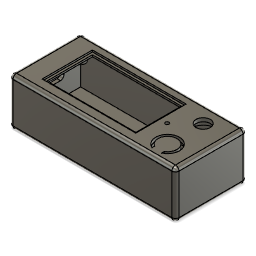
Case (Autodesk Fusion 360 design; units mm, degrees)
Autodesk Fusion 360 part; units mm, degrees
sketch "Sketch1" plane through (0, 0, 0) normal (0, 1, 0) x (1, 0, 0) in component "Toppen"
  line L0 (33.5, -15) -> (-33.5, -15)
  line L1 (-35, -13.5) -> (-35, 13.5)
  line L2 (-33.5, 15) -> (33.5, 15)
  line L3 (35, 13.5) -> (35, -13.5)
  line L4 (35, -15) -> (-35, 15) construction
  line L5 (-35, -15) -> (35, 15) construction
  arc A0 (35, 13.5) -> (33.5, 15) centre (33.5, 13.5) ccw
  arc A1 (-33.5, 15) -> (-35, 13.5) centre (-33.5, 13.5) ccw
  arc A2 (-35, -13.5) -> (-33.5, -15) centre (-33.5, -13.5) ccw
  arc A3 (33.5, -15) -> (35, -13.5) centre (33.5, -13.5) ccw
  dimension "d1" = 70
  dimension "d2" = 30
  dimension "d3" = 1.5
  constraint horizontal L0
  constraint perpendicular L0 L1
  constraint parallel L0 L2
  constraint parallel L1 L3
  constraint coincident L4 origin
  constraint coincident L5 origin
  constraint coincident L5.end L3
  constraint coincident L5.end L2
  constraint tangent L3 A0
  constraint tangent L2 A0
  constraint coincident L4.end L2
  constraint coincident L4.end L1
  constraint tangent L2 A1
  constraint tangent L1 A1
  constraint equal A0 A1
  constraint coincident L5.start L1
  constraint coincident L5.start L0
  constraint tangent L1 A2
  constraint tangent L0 A2
  constraint equal A0 A2
  constraint coincident L4.start L3
  constraint coincident L4.start L0
  constraint tangent L3 A3
  constraint tangent L0 A3
  constraint equal A0 A3
  measures "d1" distance of L4.end L5.end
  measures "d2" distance of L4.start L5.end
  measures "d3" radius of A0
extrude "Extrude1" add sketch "Sketch1" against normal blind 18.5 makes body 1 in component "Toppen"
move_body "Move1" bodies 1 to x (1, 0, 0) y (0, 1, 0) z (0, 0, 1) at (0, 15, 0) in component "Toppen"
shell "Shell1" thickness 1.5 removed faces 1 at (11.1667, -3.5, 5) on bodies 1 in component "Toppen"
extrude "Extrude1'" add sketch "Sketch1" along normal blind 1.5 separate body makes body 2 in component "Botten"
sketch "Sketch1 (2)" plane through (0, 20, 0) normal (0, 1, 0) x (-1, 0, 0) in component "Botten"
  arc A0 (35, 13.5) -> (33.5, 15) centre (33.5, 13.5) ccw
  line L0 (33.5, 15) -> (-33.5, 15)
  arc A1 (-33.5, 15) -> (-35, 13.5) centre (-33.5, 13.5) ccw
  line L1 (-35, 13.5) -> (-35, -13.5)
  arc A2 (-35, -13.5) -> (-33.5, -15) centre (-33.5, -13.5) ccw
  line L2 (-33.5, -15) -> (33.5, -15)
  arc A3 (33.5, -15) -> (35, -13.5) centre (33.5, -13.5) ccw
  line L3 (35, -13.5) -> (35, 13.5)
  line L4 (35, 0) -> (29, 0) construction
  line L5 (29, 0) -> (29, 8.75) construction
  line L6 (29, 8.75) -> (-16.7, 8.75) construction
  line L7 (-16.7, 8.75) -> (-16.7, -9.05) construction
  line L8 (-16.7, -9.05) -> (29, -9.05) construction
  line L9 (29, -9.05) -> (29, 8.75) construction
  circle A4 centre (29, -9.05) radius 2
  circle A5 centre (29, 8.75) radius 2
  circle A6 centre (-16.7, -9.05) radius 2
  circle A7 centre (-16.7, 8.75) radius 2
  line L10 (35, 0) -> (31.5, 0) construction
  line L11 (31.5, 0) -> (31.5, 11.5) construction
  line L12 (31.5, 11.5) -> (-19.5, 11.5) construction
  line L13 (-19.5, 11.5) -> (-19.5, -11.5) construction
  line L14 (-19.5, -11.5) -> (31.5, -11.5) construction
  line L15 (31.5, -11.5) -> (31.5, 11.5) construction
  line L16 (31.5, -11.5) -> (24, -11.5) construction
  line L17 (24, -11.5) -> (24, -9) construction
  line L18 (24, -9) -> (31.5, -9) construction
  line L19 (31.5, -9) -> (31.5, -11.5) construction
  line L20 (24, -9) -> (-11.5, -9) construction
  line L21 (-11.5, -9) -> (-11.5, 8.2) construction
  line L22 (-11.5, 8.2) -> (24, 8.2) construction
  line L23 (24, 8.2) -> (24, -9) construction
  line L24 (-11.5, 8.2) -> (24, -9) construction
  line L25 (-11.5, -9) -> (24, 8.2) construction
  line L26 (25, 9.2) -> (-12.5, 9.2)
  line L27 (-12.5, 9.2) -> (-12.5, -10)
  line L28 (-12.5, -10) -> (25, -10)
  line L29 (25, -10) -> (25, 9.2)
  line L30 (25, 9.2) -> (-12.5, -10) construction
  line L31 (-12.5, 9.2) -> (25, -10) construction
  line L32 (26, 10.2) -> (-13.5, 10.2)
  line L33 (-13.5, 10.2) -> (-13.5, -11)
  line L34 (-13.5, -11) -> (26, -11)
  line L35 (26, -11) -> (26, 10.2)
  line L36 (26, 10.2) -> (-13.5, -11) construction
  line L37 (-13.5, 10.2) -> (26, -11) construction
  line L38 (-16.7, -9.05) -> (-16.7, -0.05) construction
  line L39 (-16.7, -0.05) -> (-16.5, -0.05) construction
  circle A8 centre (-16.5, -0.05) radius 0.75
  point P0 (6.25, -0.4)
  point P1 (6.25, -0.4)
  dimension "d11" = 6
  dimension "d12" = 8.75
  dimension "d13" = 45.7
  dimension "d14" = 17.8
  dimension "d15" = 4
  dimension "d16" = 4
  dimension "d17" = 4
  dimension "d18" = 4
  dimension "d19" = 3.5
  dimension "d20" = 11.5
  dimension "d21" = 51
  dimension "d22" = 23
  dimension "d23" = 7.5
  dimension "d24" = 2.5
  dimension "d25" = 35.5
  dimension "d26" = 17.2
  dimension "d27" = 37.5
  dimension "d28" = 19.2
  dimension "d29" = 39.5
  dimension "d30" = 21.2
  dimension "d43" = 9
  dimension "d44" = 0.2
  dimension "d45" = 1.5
  constraint midpoint L3 L4.start
  constraint perpendicular L3 L4
  constraint perpendicular L4 L5
  constraint horizontal L6
  constraint vertical L7
  constraint horizontal L8
  constraint vertical L9
  constraint coincident L8.end L9.start
  constraint coincident L5.end L6.start
  constraint coincident L7.end L8.start
  constraint coincident L6.end L7.start
  constraint perpendicular L3 L10
  constraint perpendicular L10 L11
  constraint horizontal L12
  constraint vertical L13
  constraint horizontal L14
  constraint vertical L15
  constraint vertical L17
  constraint perpendicular L16 L17
  constraint horizontal L18
  constraint parallel L17 L19
  constraint horizontal L20
  constraint vertical L21
  constraint horizontal L22
  constraint vertical L23
  constraint horizontal L26
  constraint perpendicular L26 L27
  constraint parallel L26 L28
  constraint parallel L27 L29
  constraint coincident L30 P1
  constraint coincident L31 P1
  constraint midpoint L25 P1
  constraint horizontal L32
  constraint perpendicular L32 L33
  constraint parallel L32 L34
  constraint parallel L33 L35
  constraint coincident L36 P1
  constraint coincident L37 P1
  constraint coincident P1 P0
  constraint perpendicular L8 L38
  constraint perpendicular L38 L39
  constraint coincident L39.end A8.centre
  measures "d11" distance of L4.start L4.end
  measures "d12" distance of L4.end L5.end
  measures "d13" distance of L5.end L6.end
  measures "d14" distance of L5.end L8.end
  measures "d15" diameter of A4
  measures "d16" diameter of A5
  measures "d17" diameter of A6
  measures "d18" diameter of A7
  measures "d19" distance of L4.start L10.end
  measures "d20" distance of L10.end L11.end
  measures "d21" distance of L11.end L12.end
  measures "d22" distance of L11.end L14.end
  measures "d23" distance of L14.end L16.end
  measures "d24" distance of L14.end L18.end
  measures "d25" distance of L17.end L20.end
  measures "d26" distance of L17.end L22.end
  measures "d27" distance of L27.end L28.end
  measures "d28" distance of L26.end L27.end
  measures "d29" distance of L33.end L34.end
  measures "d30" distance of L32.end L33.end
  measures "d43" distance of L7.end L38.end
  measures "d44" distance of L38.end L39.end
  measures "d45" diameter of A8
extrude "Extrude3" cut sketch "Sketch1 (2)" against normal blind 1.5 contours L26 L27 L28 L29 sketch seen with x (1, 0, 0) y (0, 1, 0) z (0, 0, 1) at (0, -5, 0) bodies 1 in component "Toppen"
extrude "Extrude4" cut sketch "Sketch1 (2)" against normal blind 0.75 contours L32 L33 L34 L35 sketch seen with x (1, 0, 0) y (0, 1, 0) z (0, 0, 1) at (0, -5, 0) bodies 1 in component "Toppen"
extrude "Extrude5" add sketch "Sketch1 (2)" against normal blind 4.5 contours A4 | A5 | A6 | A7 sketch seen with x (1, 0, 0) y (0, 1, 0) z (0, 0, 1) at (0, -5, 0) bodies 1 in component "Toppen"
sketch "Sketch2" plane through (0, 10.5, 0) normal (0, -1, 0) x (1, 0, 0) in component "Toppen"
  circle A0 centre (-29, 8.75) radius 2
  circle A1 centre (-29, 8.75) radius 0.75
  dimension "d37" = 1.5
  constraint concentric A0 A1
  measures "d37" diameter of A1
sketch "Sketch3" plane through (0, 10.5, 0) normal (0, -1, 0) x (1, 0, 0) in component "Toppen"
  circle A0 centre (16.7, 8.75) radius 2
  circle A1 centre (16.7, 8.75) radius 0.75
  dimension "d38" = 1.5
  constraint concentric A0 A1
  measures "d38" diameter of A1
sketch "Sketch4" plane through (0, 10.5, 0) normal (0, -1, 0) x (1, 0, 0) in component "Toppen"
  circle A0 centre (16.7, -9.05) radius 2
  circle A1 centre (16.7, -9.05) radius 0.75
  dimension "d39" = 1.5
  constraint concentric A0 A1
  measures "d39" diameter of A1
sketch "Sketch5" plane through (0, 10.5, 0) normal (0, -1, 0) x (1, 0, 0) in component "Toppen"
  circle A0 centre (-29, -9.05) radius 2
  circle A1 centre (-29, -9.05) radius 0.75
  dimension "d40" = 1.5
  constraint concentric A0 A1
  measures "d40" diameter of A1
extrude "Extrude6" cut sketch "Sketch5" sketch "Sketch3" sketch "Sketch4" sketch "Sketch2" against normal blind 3 contours A1 of sketch 2 contours A1 of sketch 3 contours A1 of sketch 4 contours A1 bodies 1 in component "Toppen"
extrude "Extrude7" cut sketch "Sketch1 (2)" against normal blind 1.5 contours A8 sketch seen with x (1, 0, 0) y (0, 1, 0) z (0, 0, 1) at (0, -5, 0) bodies 1 in component "Toppen"
sketch "Sketch6" plane through (0, 15, 0) normal (0, 1, 0) x (-1, 0, 0) in component "Toppen"
  circle A0 centre (-16.5, -0.05) radius 0.75
  line L0 (-13.5, 10.2) -> (26, 10.2)
  line L1 (26, 10.2) -> (26, -11)
  line L2 (26, -11) -> (-13.5, -11)
  line L3 (-13.5, -11) -> (-13.5, 10.2)
  arc A1 (35, 13.5) -> (33.5, 15) centre (33.5, 13.5) ccw
  line L4 (33.5, 15) -> (-33.5, 15)
  arc A2 (-33.5, 15) -> (-35, 13.5) centre (-33.5, 13.5) ccw
  line L5 (-35, 13.5) -> (-35, -13.5)
  arc A3 (-35, -13.5) -> (-33.5, -15) centre (-33.5, -13.5) ccw
  line L6 (-33.5, -15) -> (33.5, -15)
  arc A4 (33.5, -15) -> (35, -13.5) centre (33.5, -13.5) ccw
  line L7 (35, -13.5) -> (35, 13.5)
  line L8 (-13.5, 10.2) -> (-13.5, 15) construction
  line L9 (-13.5, -11) -> (-13.5, -15) construction
  line L10 (-34.5607, -14.5607) -> (-13.5, 15) construction
  line L11 (-13.5, -15) -> (-34.5607, 14.5607) construction
  line L12 (-24.1868, 0) -> (-24.1868, -15) construction
  line L13 (-24.1868, 0) -> (-24.1868, 15) construction
  circle A5 centre (-24.1868, -7.5) radius 3
  circle A6 centre (-24.1868, -7.5) radius 5.5
  circle A7 centre (-24.1868, -7.5) radius 6.25
  circle A8 centre (-24.1868, 7.5) radius 5
  circle A9 centre (-24.1868, 7.5) radius 4
  line L14 (-22.1868, 12.5) -> (-26.1868, 12.5)
  line L15 (-26.1868, 12.5) -> (-26.1868, 10.5)
  line L16 (-26.1868, 10.5) -> (-22.1868, 10.5)
  line L17 (-22.1868, 10.5) -> (-22.1868, 12.5)
  line L18 (-22.1868, 12.5) -> (-26.1868, 10.5) construction
  line L19 (-26.1868, 12.5) -> (-22.1868, 10.5) construction
  point P0 (-24.1868, 11.5)
  dimension "d48" = 6
  dimension "d49" = 11
  dimension "d50" = 12.5
  dimension "d55" = 10
  dimension "d56" = 8
  dimension "d57" = 4
  dimension "d58" = 2
  constraint coincident L0.start L3.end
  constraint coincident L4 L8.end
  constraint perpendicular L4 L8
  constraint coincident L2.end L3.start
  constraint coincident L6 L9.end
  constraint perpendicular L6 L9
  constraint midpoint A3 L10.start
  constraint midpoint A2 L11.end
  constraint coincident L11 L12.start
  constraint coincident L10 L12.start
  constraint coincident L6 L12.end
  constraint perpendicular L6 L12
  constraint coincident L4 L13.end
  constraint perpendicular L4 L13
  constraint midpoint L12 A5.centre
  constraint concentric A5 A6
  constraint concentric A6 A7
  constraint midpoint L13 A8.centre
  constraint concentric A8 A9
  constraint horizontal L14
  constraint perpendicular L14 L15
  constraint parallel L14 L16
  constraint parallel L15 L17
  constraint coincident L18 P0
  constraint coincident L19 P0
  constraint coincident L13 P0
  constraint coincident A9 P0
  measures "d48" diameter of A5
  measures "d49" diameter of A6
  measures "d50" diameter of A7
  measures "d55" diameter of A8
  measures "d56" diameter of A9
  measures "d57" distance of L15.end L16.end
  measures "d58" distance of L14.end L15.end
extrude "Extrude8" cut sketch "Sketch6" against normal blind 1.5 contours A5 bodies 1 in component "Toppen"
extrude "Extrude9" add sketch "Sketch6" against normal blind 4.5 contours A7 bodies 1 in component "Toppen"
extrude "Extrude10" cut sketch "Sketch6" against normal blind 1.5 contours A8 A9 L15 L17 picked at (-26.4052, 11.5945) bodies 1 in component "Toppen"
sketch "Sketch7" plane through (0, 13.5, 0) normal (0, -1, 0) x (1, 0, 0) in component "Toppen"
  line L0 (22.1868, 12.0826) -> (22.1868, 10.9641)
  arc A0 (22.1868, 10.9641) -> (26.1868, 10.9641) centre (24.1868, 7.5) ccw
  line L1 (26.1868, 10.9641) -> (26.1868, 12.0826)
  arc A1 (22.1868, 12.0826) -> (26.1868, 12.0826) centre (24.1868, 7.5) ccw
  arc A2 (25.9368, -13.5) -> (17.9369, -7.4783) centre (24.1868, -7.5) ccw
  arc A3 (17.9369, -7.4783) -> (18.4592, -10.0014) centre (16.7, -9.05) ccw
  circle A4 centre (16.5, -0.05) radius 0.75
  circle A5 centre (-29, 8.75) radius 2
  circle A6 centre (-29, -9.05) radius 2
  circle A7 centre (16.7, 8.75) radius 2
  line L2 (-25, 9.2) -> (12.5, 9.2)
  line L3 (12.5, 9.2) -> (12.5, -10)
  line L4 (12.5, -10) -> (-25, -10)
  line L5 (-25, -10) -> (-25, 9.2)
  line L6 (33.5, 13.5) -> (-33.5, 13.5)
  line L7 (-33.5, 13.5) -> (-33.5, -13.5)
  line L8 (25.9368, -13.5) -> (33.5, -13.5)
  line L9 (33.5, -13.5) -> (33.5, 13.5)
  circle A8 centre (24.1868, 7.5) radius 2
  line L10 (-33.5, -13.5) -> (22.4368, -13.5)
  arc A9 (18.4592, -10.0014) -> (22.4368, -13.5) centre (24.1868, -7.5) ccw
  dimension "d61" = 4
  constraint concentric A0 A8
  measures "d61" diameter of A8
extrude "Extrude11" add sketch "Sketch7" along normal blind 0.6 contours A8 bodies 1 in component "Toppen"
sketch "Sketch8" plane through (-35, 0, 0) normal (-1, 0, 0) x (0, 0, 1) in component "Toppen"
  line L0 (13.5, 15) -> (-13.5, 15)
  line L1 (-13.5, 15) -> (-13.5, -3.5)
  line L2 (-13.5, -3.5) -> (13.5, -3.5)
  line L3 (13.5, -3.5) -> (13.5, 15)
  line L4 (0, 15) -> (0, 6.5) construction
  line L5 (5, 10) -> (-5, 10)
  line L6 (-6.5, 8.5) -> (-6.5, 4.5)
  line L7 (-5, 3) -> (5, 3)
  line L8 (6.5, 4.5) -> (6.5, 8.5)
  line L9 (6.5, 10) -> (-6.5, 3) construction
  line L10 (-6.5, 10) -> (6.5, 3) construction
  arc A0 (-5, 10) -> (-6.5, 8.5) centre (-5, 8.5) ccw
  arc A1 (-6.5, 4.5) -> (-5, 3) centre (-5, 4.5) ccw
  arc A2 (5, 3) -> (6.5, 4.5) centre (5, 4.5) ccw
  arc A3 (6.5, 8.5) -> (5, 10) centre (5, 8.5) ccw
  point P0 (0, 6.5)
  dimension "d64" = 8.5
  dimension "d65" = 13
  dimension "d66" = 7
  dimension "d67" = 1.5
  constraint midpoint L0 L4.start
  constraint perpendicular L0 L4
  constraint horizontal L5
  constraint perpendicular L5 L6
  constraint parallel L5 L7
  constraint parallel L6 L8
  constraint coincident L9 P0
  constraint coincident L10 P0
  constraint coincident P0 L4.end
  constraint coincident L10.start L5
  constraint coincident L10.start L6
  constraint tangent L5 A0
  constraint tangent L6 A0
  constraint coincident L9.end L7
  constraint coincident L9.end L6
  constraint tangent L7 A1
  constraint tangent L6 A1
  constraint equal A0 A1
  constraint coincident L10.end L8
  constraint coincident L10.end L7
  constraint tangent L8 A2
  constraint tangent L7 A2
  constraint equal A0 A2
  constraint coincident L9.start L5
  constraint coincident L9.start L8
  constraint tangent L5 A3
  constraint tangent L8 A3
  constraint equal A0 A3
  measures "d64" distance of L4.start P0
  measures "d65" distance of L9.end L10.end
  measures "d66" distance of L10.start L9.end
  measures "d67" radius of A0
extrude "Extrude12" cut sketch "Sketch8" against normal blind 1.5 contours L5 L6 L7 L8 A0 A1 A2 A3 bodies 1 in component "Toppen"
fillet "Fillet1" radius 1.5 8 edges at (-34.5607, 15, 14.5607) (-35, 15, 0) (-34.5607, 15, -14.5607) (0, 15, -15) (34.5607, 15, -14.5607) (35, 15, 0) (34.5607, 15, 14.5607) (0, 15, 15) on bodies 1 in component "Toppen"
fillet "Fillet1'" radius 1.5 8 edges at (-34.5607, 0, 14.5607) (-35, 0, 0) (-34.5607, 0, -14.5607) (0, 0, -15) (34.5607, 0, -14.5607) (35, 0, 0) (34.5607, 0, 14.5607) (0, 0, 15) on bodies 2 in component "Botten"
component "Botten" placed x (1, 0, 0) y (0, 1, 0) z (0, 0, 1) at (0, -5, 0)
component "Toppen" placed x (1, 0, 0) y (0, 1, 0) z (0, 0, 1) at (0, 0, 0)
equation "d1 = 51 mm + ( 2 * 2 ) * 1 mm + ( 1.5 * 2 ) * 1 mm + 10 mm + 2 mm"
equation "d2 = 23 mm + ( 2 * 2 ) * 1 mm + ( 1.5 * 2 ) * 1 mm"
equation "d4 = -15 mm - 2 mm - 1.5 mm"
equation "d11 = 2 mm + 1.5 mm + 2.5 mm"
equation "d12 = ( 17.5 / 2 ) * 1 mm"
equation "d19 = 1.5 mm + 2 mm"
equation "d20 = ( 23 / 2 ) * 1 mm"
equation "d27 = 35.5 mm + 2 mm"
equation "d28 = 17.2 mm + 2 mm"
equation "d29 = 37.5 mm + 2 mm"
equation "d30 = 19.2 mm + 2 mm"
equation "d35 = -1.5 mm - 3 mm"
equation "d50 = 11 mm + 1.5 mm"
equation "d53 = -1.5 mm - 3 mm"
equation "d64 = 1.5 mm + 3 mm + 4 mm"
